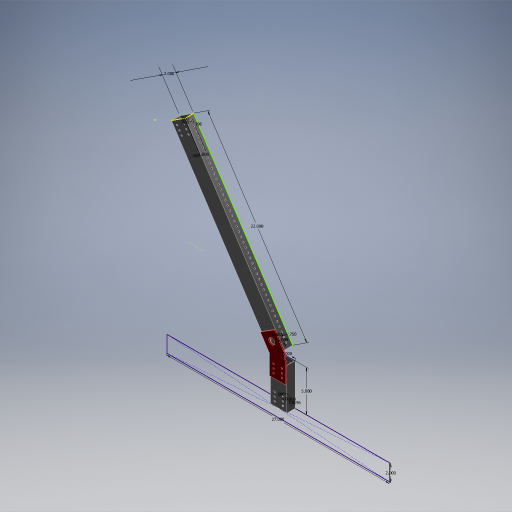
# Autodesk Inventor part: Shootaur-Superstructure
Saved by Autodesk Inventor 2024.2 (Build 282272000, 272)
## iProperties
Created: 2024-01-20
Part Number: Shootaur-Superstructure
Material: Aluminum 6061
Document SubType Name: Modeling
Designer: rohan
Density: 2.7 g/cm^3
Appearance: Aluminum - Flat
Author: rohan
Autodesk Inventor part; units mm, degrees
ref_plane "YZ Plane" through (0, 0, 0) normal (1, 0, 0) x (0, 1, 0)
ref_plane "XZ Plane" through (0, 0, 0) normal (0, 1, 0) x (-1, 0, 0)
ref_plane "XY Plane" through (0, 0, 0) normal (0, 0, 1) x (1, 0, 0)
sketch "Sketch1" plane through (0, 0, 0) normal (0, 0, 1) x (1, 0, 0)
  line L0 (-342.9, 25.4) -> (342.9, 25.4)
  line L1 (342.9, 25.4) -> (342.9, -25.4)
  line L2 (342.9, -25.4) -> (-342.9, -25.4)
  line L3 (-342.9, -25.4) -> (-342.9, 25.4)
  line L4 (-342.9, 25.4) -> (342.9, -25.4) construction
  line L5 (342.9, 25.4) -> (-342.9, -25.4) construction
  line L6 (-277.1742, 25.4) -> (-226.3742, 25.4)
  line L7 (2.2258, 25.4) -> (53.0258, 25.4)
  line L8 (53.0258, 25.4) -> (53.0258, 152.4)
  line L9 (53.0258, 152.4) -> (2.2258, 152.4)
  line L10 (2.2258, 152.4) -> (2.2258, 25.4)
  circle A0 centre (14.9258, 38.1) radius 2.4892
  circle A1 centre (40.3258, 38.1) radius 2.4892
  circle A2 centre (14.9258, 50.8) radius 2.4892
  circle A3 centre (40.3258, 50.8) radius 2.4892
  circle A4 centre (14.9258, 63.5) radius 2.4892
  circle A5 centre (40.3258, 63.5) radius 2.4892
  line L11 (-277.1742, 304.8) -> (-226.3742, 304.8) construction
  line L12 (-303.572, 629.6237) -> (-261.054, 657.424)
  line L13 (-261.054, 657.424) -> (44.749, 189.7254)
  line L14 (44.749, 189.7254) -> (2.2309, 161.9251)
  line L15 (2.2309, 161.9251) -> (-303.572, 629.6237)
  circle A6 centre (-285.9925, 625.9443) radius 2.4892
  circle A7 centre (-264.7334, 639.8444) radius 2.4892
  circle A8 centre (-279.0424, 615.3148) radius 2.4892
  circle A9 centre (-257.7834, 629.2149) radius 2.4892
  circle A10 centre (-272.0923, 604.6853) radius 2.4892
  circle A11 centre (-250.8333, 618.5854) radius 2.4892
  circle A12 centre (9.5898, 197.0843) radius 9.525
  line L16 (2.2258, 88.9) -> (53.0258, 88.9) construction
  circle A13 centre (14.9258, 139.7) radius 2.4892
  circle A14 centre (40.3258, 139.7) radius 2.4892
  circle A15 centre (14.9258, 127) radius 2.4892
  circle A16 centre (40.3258, 127) radius 2.4892
  circle A17 centre (14.9258, 114.3) radius 2.4892
  circle A18 centre (40.3258, 114.3) radius 2.4892
  point P0 (0, 0)
  point P1 (53.0258, 25.4)
  dimension "d0" = 685.8
  dimension "d1" = 50.8
  dimension "d5" = 127
  dimension "d21" = 4.9784
  dimension "d22" = 12.7
  dimension "d23" = 12.7
  dimension "d26" = 25.4
  dimension "d29" = 12.7
  dimension "d60" = 50.8
  dimension "d61" = 50.8
  dimension "d62" = 4.9784
  dimension "d63" = 12.7
  dimension "d64" = 12.7
  dimension "d67" = 25.4
  dimension "d70" = 12.7
  dimension "d73" = 19.05
  dimension "d74" = 25.4
  dimension "d75" = 25.4
  dimension "d87" = 558.8
  constraints: 34 end point, 19 centre point, 6 parallel, 6 symmetric about line, 4 horizontal, 4 midpoint, 3 perpendicular, 2 point on line, 1 vertical, 28 other
  measures "d0" distance of L1.end L2.end
  measures "d1" distance of L0.end L1.end
  measures "d5" distance of L8.end L7.end
  measures "d21" diameter of A0
  measures "d22" distance from line of L10 A0.centre
  measures "d23" distance from line of A0.centre L0
  measures "d26" distance of A0.centre A1.centre
  measures "d29" distance of A0.centre A2.centre
  measures "d60" distance of L12.start L12.end
  measures "d61" distance of L8.end L9.end
  measures "d62" diameter of A6
  measures "d63" distance from line of A6.centre L12
  measures "d64" distance from line of L15 A6.centre
  measures "d67" distance of A6.centre A7.centre
  measures "d70" distance of A6.centre A8.centre
  measures "d73" diameter of A12
  measures "d74" distance from line of A12.centre L15
  measures "d75" distance from line of A12.centre L14
  measures "d87" distance of L12.end L13.end
extrude "Extrusion8" add sketch "Sketch1" along normal blind 25.4 contours L12 L13 L14 L15
extrude "Extrusion9" add sketch "Sketch1" along normal blind 25.4 separate body contours L10 L9 L8 L0
sketch "Sketch7" plane through (0, 0, 25.4) normal (0, 0, 1) x (1, 0, 0)
  line L0 (2.2309, 161.9251) -> (44.749, 189.7254) projected
  line L1 (44.749, 189.7254) -> (-261.054, 657.424) projected
  line L2 (-261.054, 657.424) -> (-303.572, 629.6237) projected
  line L3 (-303.572, 629.6237) -> (2.2309, 161.9251) projected
  circle A0 centre (9.5898, 197.0843) radius 9.525 projected
  circle A1 centre (-250.8333, 618.5854) radius 2.4892 projected
  circle A2 centre (-272.0923, 604.6853) radius 2.4892 projected
  circle A3 centre (-257.7834, 629.2149) radius 2.4892 projected
  circle A4 centre (-279.0424, 615.3148) radius 2.4892 projected
  circle A5 centre (-264.7334, 639.8444) radius 2.4892 projected
  circle A6 centre (-285.9925, 625.9443) radius 2.4892 projected
  line L4 (2.2258, 152.4) -> (2.2258, 25.4) projected
  line L5 (2.2258, 25.4) -> (53.0258, 25.4) projected
  line L6 (53.0258, 25.4) -> (53.0258, 152.4) projected
  line L7 (53.0258, 152.4) -> (2.2258, 152.4) projected
  circle A7 centre (40.3258, 139.7) radius 2.4892 projected
  circle A8 centre (40.3258, 114.3) radius 2.4892 projected
  circle A9 centre (14.9258, 127) radius 2.4892 projected
  circle A10 centre (14.9258, 38.1) radius 2.4892 projected
  circle A11 centre (40.3258, 38.1) radius 2.4892 projected
  circle A12 centre (14.9258, 50.8) radius 2.4892 projected
  circle A13 centre (40.3258, 50.8) radius 2.4892 projected
  circle A14 centre (14.9258, 63.5) radius 2.4892 projected
  circle A15 centre (40.3258, 63.5) radius 2.4892 projected
  circle A16 centre (40.3258, 127) radius 2.4892 projected
  circle A17 centre (14.9258, 114.3) radius 2.4892 projected
  circle A18 centre (14.9258, 139.7) radius 2.4892 projected
  line L8 (2.2258, 152.4) -> (2.2309, 161.9251)
  line L9 (2.2309, 161.9251) -> (-25.5694, 204.4432)
  line L10 (-303.572, 629.6237) -> (2.2309, 161.9251) projected
  line L11 (-25.5694, 204.4432) -> (17.415, 231.5303)
  line L12 (17.415, 231.5303) -> (44.749, 189.7254)
  line L13 (44.749, 189.7254) -> (53.0258, 152.4)
  line L14 (53.0258, 152.4) -> (53.0258, 101.6)
  line L15 (53.0258, 25.4) -> (53.0258, 152.4) projected
  line L16 (53.0258, 101.6) -> (2.2258, 101.6)
  line L17 (2.2258, 152.4) -> (2.2258, 25.4) projected
  line L18 (2.2258, 101.6) -> (2.2258, 152.4)
  point P0 (0, 0)
  dimension "d80" = 50.8
  dimension "d81" = 50.8
  constraints: 16 end point, 4 point on line, 2 perpendicular, 1 collinear
  measures "d80" distance of L0.start L9.end
  measures "d81" distance of L6.end L14.end
extrude "Extrusion10" add sketch "Sketch7" along normal blind 3.175 separate body contours L3 L11 L1 L0 | L0 L13 L7 L8 | L7 L6 L16 L4
sketch "Sketch8" plane through (2.2258, 152.4, 0) normal (0, 1, 0) x (1, 0, 0)
  line L0 (50.8, 0) -> (0, 0) projected
  line L1 (0, 0) -> (0, -25.4) projected
  line L2 (50.8, -25.4) -> (0, -25.4) projected
  line L3 (50.8, 0) -> (50.8, -25.4) projected
  line L4 (1.5875, -1.5875) -> (49.2125, -1.5875)
  line L5 (49.2125, -1.5875) -> (49.2125, -23.8125)
  line L6 (49.2125, -23.8125) -> (1.5875, -23.8125)
  line L7 (1.5875, -23.8125) -> (1.5875, -1.5875)
  point P0 (-2.2258, 0)
  dimension "d84" = 1.5875
  constraints: 8 end point, 3 other
  measures "d84" distance between parallel lines of L0 L4
extrude "Extrusion11" cut sketch "Sketch8" against normal blind 209.55 contours L4 L5 L6 L7 bodies 2
sketch "Sketch9" plane through (-303.572, 629.6237, 25.4) normal (-0.5472494, 0.8369696, 0) x (0.8369696, 0.5472494, 0)
  line L0 (50.8, 25.4) -> (0, 25.4) projected
  line L1 (0, 25.4) -> (0, 0) projected
  line L2 (50.8, 0) -> (0, 0) projected
  line L3 (50.8, 25.4) -> (50.8, 0) projected
  point P0 (-90.4806, 25.4)
sketch "Sketch10" plane through (-303.572, 629.6237, 25.4) normal (-0.5472494, 0.8369696, 0) x (0.8369696, 0.5472494, 0)
  line L0 (50.8, 25.4) -> (0, 25.4) projected
  line L1 (0, 25.4) -> (0, 0) projected
  line L2 (50.8, 0) -> (0, 0) projected
  line L3 (50.8, 25.4) -> (50.8, 0) projected
  line L4 (1.5875, 1.5875) -> (1.5875, 23.8125)
  line L5 (1.5875, 23.8125) -> (49.2125, 23.8125)
  line L6 (49.2125, 23.8125) -> (49.2125, 1.5875)
  line L7 (49.2125, 1.5875) -> (1.5875, 1.5875)
  point P0 (-90.4806, 25.4)
  dimension "d88" = 1.5875
  constraints: 8 end point, 3 other
  measures "d88" distance between parallel lines of L1 L4
extrude "Extrusion12" cut sketch "Sketch10" against normal up to surface (558.8 mm away) contours L4 L5 L6 L7 bodies 1
sketch "Sketch11" plane through (-261.054, 657.424, 25.4) normal (0.8369696, 0.5472494, 0) x (0, 0, -1)
  circle A0 centre (12.7, -12.7) radius 2.4892
  line L0 (25.4, 0) -> (0, 0) projected
  line L1 (0, -558.8) -> (0, 0) projected
  circle A1 centre (12.7, -25.4) radius 2.4892
  circle A2 centre (12.7, -38.1) radius 2.4892
  circle A3 centre (12.7, -50.8) radius 2.4892
  circle A4 centre (12.7, -63.5) radius 2.4892
  circle A5 centre (12.7, -76.2) radius 2.4892
  circle A6 centre (12.7, -88.9) radius 2.4892
  circle A7 centre (12.7, -101.6) radius 2.4892
  circle A8 centre (12.7, -114.3) radius 2.4892
  circle A9 centre (12.7, -127) radius 2.4892
  circle A10 centre (12.7, -139.7) radius 2.4892
  circle A11 centre (12.7, -152.4) radius 2.4892
  circle A12 centre (12.7, -165.1) radius 2.4892
  circle A13 centre (12.7, -177.8) radius 2.4892
  circle A14 centre (12.7, -190.5) radius 2.4892
  circle A15 centre (12.7, -203.2) radius 2.4892
  circle A16 centre (12.7, -215.9) radius 2.4892
  circle A17 centre (12.7, -228.6) radius 2.4892
  circle A18 centre (12.7, -241.3) radius 2.4892
  circle A19 centre (12.7, -254) radius 2.4892
  circle A20 centre (12.7, -266.7) radius 2.4892
  circle A21 centre (12.7, -279.4) radius 2.4892
  circle A22 centre (12.7, -292.1) radius 2.4892
  circle A23 centre (12.7, -304.8) radius 2.4892
  circle A24 centre (12.7, -317.5) radius 2.4892
  circle A25 centre (12.7, -330.2) radius 2.4892
  circle A26 centre (12.7, -342.9) radius 2.4892
  circle A27 centre (12.7, -355.6) radius 2.4892
  circle A28 centre (12.7, -368.3) radius 2.4892
  circle A29 centre (12.7, -381) radius 2.4892
  circle A30 centre (12.7, -393.7) radius 2.4892
  circle A31 centre (12.7, -406.4) radius 2.4892
  circle A32 centre (12.7, -419.1) radius 2.4892
  circle A33 centre (12.7, -431.8) radius 2.4892
  circle A34 centre (12.7, -444.5) radius 2.4892
  circle A35 centre (12.7, -457.2) radius 2.4892
  circle A36 centre (12.7, -469.9) radius 2.4892
  circle A37 centre (12.7, -482.6) radius 2.4892
  circle A38 centre (12.7, -495.3) radius 2.4892
  circle A39 centre (12.7, -508) radius 2.4892
  circle A40 centre (12.7, -520.7) radius 2.4892
  circle A41 centre (12.7, -533.4) radius 2.4892
  circle A42 centre (12.7, -546.1) radius 2.4892
  point P0 (25.4, -693.1055)
  dimension "d91" = 4.9784
  dimension "d92" = 12.7
  dimension "d93" = 12.7
  dimension "d96" = 12.7
  constraints: 43 centre point, 1 vertical, 84 other
  measures "d91" diameter of A0
  measures "d92" distance from line of L0 A0.centre
  measures "d93" distance from line of L1 A0.centre
  measures "d96" distance of A0.centre A1.centre
extrude "Extrusion13" cut sketch "Sketch11" against normal blind 125.7808 bodies 1
